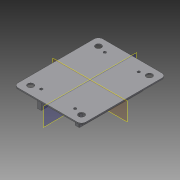
# Autodesk Inventor part: amorti
Saved by Autodesk Inventor 2015 (Build 190159000, 159)
## iProperties
Created: 2015-02-17
Part Number: amorti
Material: Generic
Document SubType Name: Modeling
Designer: Piotr
Density: 1 g/cm^3
Appearance: Default
Mass: 30.9917 g
Surface Area: 261.975 cm^2
Volume: 30.9917 cm^3
Author: Piotr
Autodesk Inventor part; units mm, degrees
ref_plane "YZ Plane" through (0, 0, 0) normal (1, 0, 0) x (0, 1, 0)
ref_plane "XZ Plane" through (0, 0, 0) normal (0, 1, 0) x (-1, 0, 0)
ref_plane "XY Plane" through (0, 0, 0) normal (0, 0, 1) x (1, 0, 0)
sketch "Sketch1" plane through (0, 0, 0) normal (0, 0, 1) x (1, 0, 0)
  line L0 (-40, -50) -> (40, -50)
  line L1 (40, -50) -> (40, 50)
  line L2 (40, 50) -> (-40, 50)
  line L3 (-40, 50) -> (-40, -50)
  line L4 (-40, -50) -> (40, 50) construction
  line L5 (40, -50) -> (-40, 50) construction
  point P0 (0, 0)
  dimension "d0" = 80
  dimension "d1" = 100
  constraints: 12 end point, 2 midpoint, 2 parallel, 1 horizontal, 1 perpendicular
  measures "d0" distance of L1.end L2.end
  measures "d1" distance of L0.end L1.end
extrude "Extrusion1" add sketch "Sketch1" along normal blind 1.5
fillet "Fillet1" radius 5 1 edges at (40, 50, 0.75)
fillet "Fillet1" radius 5 3 edges at (-40, -50, 0.75) (40, -50, 0.75) (-40, 50, 0.75)
sketch "Sketch2" plane through (0, 0, 0) normal (0, 0, -1) x (-1, 0, 0)
  line L0 (30, 40) -> (-30, 40) construction
  line L1 (-30, 40) -> (-30, -40) construction
  line L2 (-30, -40) -> (30, -40) construction
  line L3 (30, -40) -> (30, 40) construction
  line L4 (30, 40) -> (-30, -40) construction
  line L5 (-30, 40) -> (30, -40) construction
  circle A0 centre (30, -40) radius 3.5
  point P0 (0, 0)
  dimension "d6" = 60
  dimension "d7" = 80
  dimension "d8" = 7
  constraints: 12 end point, 2 midpoint, 2 parallel, 1 centre point, 1 coincident, 1 horizontal, 1 perpendicular
  measures "d6" distance of L1.end L2.end
  measures "d7" distance of L0.end L1.end
  measures "d8" diameter of A0
extrude "Extrusion2" cut sketch "Sketch2" against normal through all
mirror "Mirror1" about plane through (0, 0, 0) normal (0, 1, 0) of "Extrusion2"
mirror "Mirror2" about plane through (0, 0, 0) normal (1, 0, 0) of "Extrusion2", "Mirror1"
sketch "Sketch3" plane through (0, 0, 0) normal (0, 0, -1) x (-1, 0, 0)
  line L0 (22.5, -40) -> (-22.5, -40)
  line L1 (-22.5, -40) -> (-22.5, 40)
  line L2 (-22.5, 40) -> (22.5, 40)
  line L3 (22.5, 40) -> (22.5, -40)
  line L4 (22.5, -40) -> (-22.5, 40) construction
  line L5 (-22.5, -40) -> (22.5, 40) construction
  point P0 (0, 0)
  dimension "d11" = 45
  dimension "d12" = 80
  constraints: 12 end point, 2 midpoint, 2 parallel, 1 horizontal, 1 perpendicular
  measures "d11" distance of L0.start L0.end
  measures "d12" distance of L0.end L1.end
extrude "Extrusion3" add sketch "Sketch3" along normal blind 18
sketch "Sketch4" plane through (0, 0, -18) normal (0, 0, -1) x (-1, 0, 0)
  line L0 (17.5, -35) -> (-17.5, -35)
  line L1 (-17.5, -35) -> (-17.5, 35)
  line L2 (-17.5, 35) -> (17.5, 35)
  line L3 (17.5, 35) -> (17.5, -35)
  line L4 (17.5, -35) -> (-17.5, 35) construction
  line L5 (-17.5, -35) -> (17.5, 35) construction
  point P0 (0, 0)
  dimension "d15" = 35
  dimension "d16" = 70
  constraints: 12 end point, 2 midpoint, 2 parallel, 1 horizontal, 1 perpendicular
  measures "d15" distance of L0.start L0.end
  measures "d16" distance of L0.end L1.end
extrude "Extrusion4" cut sketch "Sketch4" against normal blind 18
sketch "Sketch6" plane through (0, 0, -18) normal (0, 0, -1) x (-1, 0, 0)
  line L0 (17.5, -35) -> (-17.5, -35) construction
  line L1 (-22.5, -40) -> (22.5, -40) construction
  line L2 (-17.5, -35) -> (17.5, -35)
  line L3 (17.5, -35) -> (17.5, -40)
  line L4 (17.5, -40) -> (-17.5, -40)
  line L5 (-17.5, -40) -> (-17.5, -35)
  point P0 (0, 0)
  constraints: 8 end point, 2 parallel, 1 horizontal, 1 perpendicular, 1 point on line
extrude "Extrusion6" cut sketch "Sketch6" against normal blind 18
sketch "Sketch7" plane through (0, 0, -18) normal (0, 0, -1) x (-1, 0, 0)
  line L0 (-17.5, -40) -> (-17.5, 35) projected
  line L1 (-22.5, -40) -> (-17.5, -40)
  line L2 (-17.5, -40) -> (-17.5, -35)
  line L3 (-17.5, -35) -> (-22.5, -35)
  line L4 (-22.5, -35) -> (-22.5, -40)
  point P0 (0, 0)
  dimension "d27" = 5
  constraints: 8 end point, 2 parallel, 1 horizontal, 1 perpendicular, 1 point on line
  measures "d27" distance of L3.end L1.start
extrude "Extrusion7" cut sketch "Sketch7" against normal blind 18
sketch "Sketch8" plane through (0, 0, -18) normal (0, 0, -1) x (-1, 0, 0)
  line L0 (17.5, -40) -> (22.5, -40) projected
  line L1 (17.5, 35) -> (17.5, -40) projected
  point P0 (0, 0)
  point P1 (20, -37.5)
  dimension "d30" = 2.5
  dimension "d31" = 2.5
  measures "d30" distance from line of L0 point (20, -37.5)
  measures "d31" distance from line of point (20, -37.5) L1
hole "Hole1" at (-20, -37.5, -18) direction (0, 0, 1) diameter 3.1 end through all
mirror "Mirror3" about plane through (0, 0, 0) normal (0, 1, 0) of "Hole1"
mirror "Mirror4" about plane through (0, 0, 0) normal (1, 0, 0) of "Hole1", "Mirror3"
ref_plane "Work Plane1" through (-22.5, 0, -18) normal (0, -1, 0) x (1, 0, 0)
sketch "Sketch9" plane through (-22.5, 0, -18) normal (0, -1, 0) x (1, 0, 0)
  line L0 (0, 0) -> (-0.7213, 10.6827) construction
  line L1 (-0.7213, 10.6827) -> (-17.5, 18) construction
  spline S0 degree 2 poles (0, 0) (-0.7213, 10.6827) (-17.5, 18) knots 1 1 1 2 2 2
  point P0 (22.5, 18)
  constraints: 3 other
extrude "Rib1" add sketch "Sketch9" along normal mid plane 2 rib yes fills toward (-4.6998, 9.8762) open curves S0
pattern_linear "Rectangular Pattern1" count 5 spacing 15 along (0, 1, 0) of "Rib1" first direction both ways yes
mirror "Mirror5" about plane through (0, 0, 0) normal (1, 0, 0) of "Rib1", "Rectangular Pattern1"
ref_plane "Work Plane2" through (0, 40, -18) normal (-1, 0, 0) x (0, 0, 1)
sketch "Sketch10" plane through (0, 40, -18) normal (-1, 0, 0) x (0, 0, 1)
  line L0 (0, 0) -> (9.5236, 0.6456) construction
  line L1 (9.5236, 0.6456) -> (18, 10) construction
  spline S0 degree 2 poles (0, 0) (9.5236, 0.6456) (18, 10) knots 1 1 1 2 2 2
  point P0 (18, -40)
  constraints: 3 other
extrude "Rib2" add sketch "Sketch10" along normal mid plane 2 rib yes fills toward (9.2861, 2.7791) open curves S0
pattern_linear "Rectangular Pattern2" count 5 spacing 10 along (-1, 0, 0) of "Rib2" first direction both ways yes
fillet "Fillet5" radius 0.5 4 edges at (22.5, 40, -9) (-22.5, 40, -9) (22.5, -35, -9) (-22.5, -40, -9)
body "Solid1"
